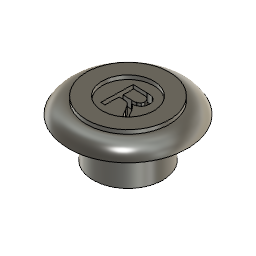
Ensamble Desafío 1 V2 (Autodesk Fusion 360 archive; units mm, degrees)
design "Tapon"
Autodesk Fusion 360 part; units mm, degrees
sketch "Boceto1" plane through (0, 0, 0) normal (0, 0, 1) x (1, 0, 0)
  circle A0 centre (0, 0) radius 4.4
  circle A1 centre (0, 0) radius 3.25
  dimension "d1" = 8.8
  dimension "d2" = 6.5
  constraint coincident A0.centre A1.centre
  constraint concentric A0 A1
  measures "d1" diameter of A0
  measures "d2" diameter of A1
extrude "Extruir1" add sketch "Boceto1" along normal blind 5 makes body 1
sketch "Boceto2" plane through (0, 0, 5) normal (0, 0, 1) x (-1, 0, 0)
  circle A0 centre (0, 0) radius 3.25
  circle A1 centre (0, 0) radius 4.4
  circle A2 centre (0, 0) radius 7.5
  dimension "d5" = 15
  constraint coincident A0.centre A1.centre
  measures "d5" diameter of A2
extrude "Extruir2" add sketch "Boceto2" along normal blind 1.5 separate body makes body 2 at (-0.0595, -0.9382, 5) makes body 3 at (-6.4224, 0.5912, 5)
fillet "Empalme1" radius 2.5 1 edges at (6.9925, 2.7121, 6.5) on bodies 3
sketch "Boceto3" plane through (0, 0, 6.5) normal (0, 0, 1) x (-1, 0, 0)
  circle A0 centre (0, 0) radius 3.25
  line L0 (1.8776, -1.4222) -> (-0.8068, -1.3612) construction
  line L1 (-0.8068, -1.3612) -> (-0.8459, -3.0856) construction
  line L2 (-0.8459, -3.0856) -> (1.8384, -3.1465) construction
  line L3 (1.8384, -3.1465) -> (1.8776, -1.4222) construction
  dimension "d10" = 4
  text T0 "R" font "Arial" height 4 align left top in box 2.685 x 1.7248 at (1.8776, -1.4222) x (-0.999742, 0.022695) y (-0.022695, -0.999742) spacing 1 kerned
extrude "Extruir3" cut sketch "Boceto3" against normal blind 1 text T0 bodies 2
extrude "Extruir4" add 1 faces at (4.0003, -0.2186, 5) along direction (0, 0, 1) blind 2 on bodies 1 bodies 1 2 3
extrude "Extruir5" add 1 faces at (0.976, 0.965, 5) along direction (0, 0, -1) blind 5 on bodies 1 bodies 1
extrude "Extruir6" add 1 faces at (4.9197, -0.2588, 6.5) along direction (0, 0, 1) blind 0.5 on bodies 1 bodies 1
equation "d11 = 'R'"
